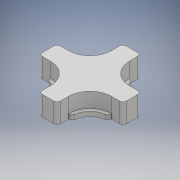
# Autodesk Inventor part: Groboy Buttons D-Pad
Saved by Autodesk Inventor 2017 SP1 (Build 210196100, 196)
## iProperties
Created: 2017-10-10
Part Number: Groboy Buttons D-Pad
Material: Generic
Document SubType Name: Modeling
Designer: Groguard
Density: 1 g/cm^3
Appearance: Default
Author: Groguard
Autodesk Inventor part; units mm, degrees
ref_plane "YZ Plane" through (0, 0, 0) normal (1, 0, 0) x (0, 1, 0)
ref_plane "XZ Plane" through (0, 0, 0) normal (0, 1, 0) x (-1, 0, 0)
ref_plane "XY Plane" through (0, 0, 0) normal (0, 0, 1) x (1, 0, 0)
sketch "Sketch1" plane through (0, 0, 0) normal (0, 0, 1) x (1, 0, 0)
  line L0 (50.75, 32.3006) -> (46.25, 32.3006)
  line L1 (46.25, 32.3006) -> (46.25, 39.8006)
  line L2 (46.25, 39.8006) -> (50.75, 39.8006)
  arc A0 (50.75, 39.8006) -> (56.25, 45.3006) centre (50.75, 45.3006) ccw
  line L3 (56.25, 45.3006) -> (56.25, 49.8006)
  line L4 (56.25, 49.8006) -> (63.75, 49.8006)
  line L5 (63.75, 49.8006) -> (63.75, 45.3006)
  arc A1 (63.75, 45.3006) -> (69.2516, 39.8006) centre (69.25, 45.3006) ccw
  line L6 (69.2516, 39.8006) -> (73.7503, 39.8165)
  line L7 (73.7503, 39.8165) -> (73.7589, 32.3006)
  line L8 (73.7589, 32.3006) -> (69.25, 32.3006)
  arc A2 (69.25, 32.3006) -> (63.75, 26.8006) centre (69.25, 26.8006) ccw
  line L9 (63.75, 26.8006) -> (63.75, 22.3006)
  line L10 (63.75, 22.3006) -> (56.25, 22.3006)
  line L11 (56.25, 22.3006) -> (56.25, 26.8006)
  arc A3 (56.25, 26.8006) -> (50.75, 32.3006) centre (50.75, 26.8006) ccw
  line L12 (47.25, 33.3006) -> (50.75, 33.3006)
  arc A4 (57.25, 26.8006) -> (50.75, 33.3006) centre (50.75, 26.8006) ccw
  line L13 (57.25, 26.8006) -> (57.25, 23.3006)
  line L14 (57.25, 23.3006) -> (62.75, 23.3006)
  line L15 (62.75, 23.3006) -> (62.75, 26.8006)
  arc A5 (69.25, 33.3006) -> (62.75, 26.8006) centre (69.25, 26.8006) ccw
  line L16 (69.25, 33.3006) -> (72.7578, 33.3006)
  line L17 (72.7578, 33.3006) -> (72.7514, 38.813)
  line L18 (72.7514, 38.813) -> (69.2535, 38.8006)
  arc A6 (62.75, 45.3006) -> (69.2535, 38.8006) centre (69.25, 45.3006) ccw
  line L19 (62.75, 45.3006) -> (62.75, 48.8006)
  line L20 (62.75, 48.8006) -> (57.25, 48.8006)
  line L21 (57.25, 48.8006) -> (57.25, 45.3006)
  arc A7 (50.75, 38.8006) -> (57.25, 45.3006) centre (50.75, 45.3006) ccw
  line L22 (50.75, 38.8006) -> (47.25, 38.8006)
  line L23 (47.25, 38.8006) -> (47.25, 33.3006)
  point P0 (0, 0)
  dimension "d47" = 1
  constraints: 48 end point, 16 point on circle, 8 centre point, 15 other
  measures "d47" distance between parallel lines of L0 L12
extrude "Extrusion1" add sketch "Sketch1" along normal blind 6 contours L0 L1 L2 A0 L3 L4 L5 A1 L6 L7 L8 A2 L9 L10 L11 A3 | L23 L22 A7 L21 L20 L19 A6 L18 L17 L16 A5 L15 L14 L13 A4 L12
sketch "Sketch2" plane through (0, 0, 6) normal (0, 0, 1) x (1, 0, 0)
  line L0 (50.75, 32.3006) -> (46.25, 32.3006)
  line L1 (46.25, 32.3006) -> (46.25, 39.8006)
  line L2 (46.25, 39.8006) -> (50.75, 39.8006)
  arc A0 (50.75, 39.8006) -> (56.25, 45.3006) centre (50.75, 45.3006) ccw
  line L3 (56.25, 49.8006) -> (63.75, 49.8006)
  line L4 (63.75, 49.8006) -> (63.75, 45.3006)
  arc A1 (63.75, 45.3006) -> (69.2516, 39.8006) centre (69.25, 45.3006) ccw
  line L5 (69.2516, 39.8006) -> (73.7498, 39.8006)
  line L6 (73.7498, 39.8006) -> (73.732, 32.3006)
  line L7 (73.732, 32.3006) -> (69.25, 32.3006)
  arc A2 (69.25, 32.3006) -> (63.75, 26.8006) centre (69.25, 26.8006) ccw
  line L8 (63.75, 26.8006) -> (63.75, 22.3006)
  line L9 (63.75, 22.3006) -> (56.25, 22.3006)
  line L10 (56.25, 22.3006) -> (56.25, 26.8006)
  arc A3 (56.25, 26.8006) -> (50.75, 32.3006) centre (50.75, 26.8006) ccw
  line L11 (47.25, 33.3006) -> (50.75, 33.3006)
  arc A4 (57.25, 26.8006) -> (50.75, 33.3006) centre (50.75, 26.8006) ccw
  line L12 (57.25, 26.8006) -> (57.25, 23.3006)
  line L13 (57.25, 23.3006) -> (62.75, 23.3006)
  line L14 (62.75, 23.3006) -> (62.75, 26.8006)
  arc A5 (69.25, 33.3006) -> (62.75, 26.8006) centre (69.25, 26.8006) ccw
  line L15 (69.25, 33.3006) -> (72.7343, 33.3006)
  line L16 (72.7343, 33.3006) -> (72.7474, 38.8006)
  line L17 (72.7474, 38.8006) -> (69.2516, 38.8006)
  arc A6 (62.75, 45.3006) -> (69.2516, 38.8006) centre (69.25, 45.3006) ccw
  line L18 (62.75, 45.3006) -> (62.75, 48.8006)
  line L19 (62.75, 48.8006) -> (57.25, 48.8006)
  line L20 (57.25, 48.8006) -> (57.25, 45.3006)
  arc A7 (50.75, 38.8006) -> (57.25, 45.3006) centre (50.75, 45.3006) ccw
  line L21 (50.75, 38.8006) -> (47.25, 38.8006)
  line L22 (47.25, 38.8006) -> (47.25, 33.3006)
  line L23 (50.75, 33.3006) -> (50.75, 32.3006)
  line L24 (50.75, 38.8006) -> (50.75, 39.8006)
  line L25 (56.25, 49.8006) -> (56.25, 45.3006)
  line L26 (56.25, 45.3006) -> (57.25, 45.3006)
  line L27 (62.75, 45.3006) -> (63.75, 45.3006)
  line L28 (69.2516, 38.8006) -> (69.2516, 39.8006)
  line L29 (69.25, 33.3006) -> (69.25, 32.3006)
  line L30 (62.75, 26.8006) -> (63.75, 26.8006)
  line L31 (56.25, 26.8006) -> (56.25, 22.3006) projected
  line L32 (56.25, 26.8006) -> (57.25, 26.8006)
  dimension "d48" = 1
  constraints: 64 end point, 16 point on circle, 8 centre point, 4 vertical, 2 perpendicular, 1 horizontal, 11 other
  measures "d48" distance between parallel lines of L0 L11
sketch "Sketch4" plane through (0, 0, 0) normal (0, 0, -1) x (-1, 0, 0)
  line L0 (-73.75, 32.3006) -> (-73.75, 39.8006) projected
  line L1 (-73.75, 36.0506) -> (-46.25, 36.0506)
  line L2 (-46.25, 39.8006) -> (-46.25, 32.3006) projected
  circle A0 centre (-60, 36.0506) radius 3
  point P0 (0, 0)
  dimension "d31" = 6
  constraints: 3 midpoint, 2 end point, 1 centre point
  measures "d31" diameter of A0
extrude "Extrusion4" add sketch "Sketch4" along normal blind 2.7
fillet "Fillet4" radius 2 1 edges at (63, 36.0506, -2.7)
extrude "Extrusion7" cut sketch "Sketch2" against normal blind 4.6 contours L23 A4 L32 A3 | A0 L26 A7 L24 | L30 A5 L29 A2 | A1 L28 A6 L27
sketch "Sketch5" plane through (0, 0, 6) normal (0, 0, 1) x (1, 0, 0)
  line L0 (62.75, 23.3006) -> (62.75, 26.8006)
  line L1 (63.75, 26.8006) -> (63.75, 22.3006)
  line L2 (57.25, 26.8006) -> (57.25, 23.3006)
  line L3 (57.25, 23.3006) -> (62.75, 23.3006)
  line L4 (56.25, 22.3006) -> (56.25, 26.8006)
  line L5 (63.75, 22.3006) -> (56.25, 22.3006)
  line L6 (56.25, 49.8006) -> (63.75, 49.8006)
  line L7 (63.75, 49.8006) -> (63.75, 45.3006)
  line L8 (57.25, 48.8006) -> (57.25, 45.3006)
  line L9 (62.75, 48.8006) -> (57.25, 48.8006)
  line L10 (62.75, 45.3006) -> (62.75, 48.8006)
  line L11 (50.75, 32.3006) -> (46.25, 32.3006)
  line L12 (46.25, 32.3006) -> (46.25, 39.8006)
  line L13 (46.25, 39.8006) -> (50.75, 39.8006)
  line L14 (47.25, 33.3006) -> (50.75, 33.3006)
  line L15 (47.25, 38.8006) -> (47.25, 33.3006)
  line L16 (50.75, 38.8006) -> (47.25, 38.8006)
  line L17 (50.75, 33.3006) -> (50.75, 32.3006)
  line L18 (50.75, 38.8006) -> (50.75, 39.8006)
  line L19 (56.25, 49.8006) -> (56.25, 45.3006)
  line L20 (56.25, 45.3006) -> (57.25, 45.3006)
  line L21 (62.75, 45.3006) -> (63.75, 45.3006)
  line L22 (62.75, 26.8006) -> (63.75, 26.8006)
  line L23 (56.25, 26.8006) -> (56.25, 22.3006)
  line L24 (56.25, 26.8006) -> (57.25, 26.8006)
  line L25 (73.7589, 32.3006) -> (69.25, 32.3006) projected
  line L26 (69.25, 32.3006) -> (73.7589, 32.3006)
  line L27 (73.7589, 32.3006) -> (73.7503, 39.8165) projected
  line L28 (73.7589, 32.3006) -> (73.7503, 39.8165)
  line L29 (69.2516, 39.8006) -> (73.7503, 39.8165) projected
  line L30 (73.7503, 39.8165) -> (69.2516, 39.8006)
  line L31 (69.2516, 39.8006) -> (69.2516, 38.8006) projected
  line L32 (69.2516, 39.8006) -> (69.2516, 38.8006)
  line L33 (69.25, 33.3006) -> (69.25, 32.3006) projected
  line L34 (69.25, 32.3006) -> (69.25, 33.3006)
  line L35 (69.25, 33.3006) -> (72.7582, 33.3006)
  line L36 (72.7582, 33.3006) -> (72.7582, 38.8006)
  line L37 (72.7582, 38.8006) -> (69.2516, 38.8006)
  point P0 (0, 0)
  point P1 (50.75, 26.8006)
  dimension "d51" = 1
  constraints: 66 end point, 5 collinear, 4 perpendicular, 2 horizontal, 2 vertical, 3 other
  measures "d51" distance between parallel lines of L11 L14
extrude "Extrusion8" cut sketch "Sketch5" against normal blind 6
fillet "Fillet6" radius 1 8 edges at (72.7582, 33.3006, 3) (72.7582, 38.8006, 3) (62.75, 23.3006, 3) (57.25, 23.3006, 3) (62.75, 48.8006, 3) (57.25, 48.8006, 3) (47.25, 38.8006, 3) (47.25, 33.3006, 3)
fillet "Fillet7" radius 1 8 edges at (69.25, 32.3006, 0.7) (63.75, 26.8006, 0.7) (69.2516, 39.8006, 0.7) (63.75, 45.3006, 0.7) (56.25, 26.8006, 0.7) (50.75, 32.3006, 0.7) (56.25, 45.3006, 0.7) (50.75, 39.8006, 0.7)
body "Solid1"
